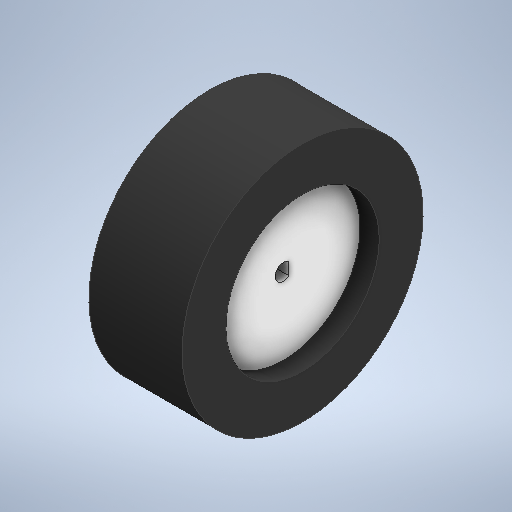
# Autodesk Inventor part: llanta
Saved by Autodesk Inventor 2025.2 (Build 292293000, 293)
## iProperties
Created: 2025-06-11
Part Number: llanta
Material: Generic
Document SubType Name: Modeling
Designer: cdavi
Density: 1 g/cm^3
Appearance: Default
Author: cdavi
Autodesk Inventor part; units mm, degrees
ref_plane "YZ Plane" through (0, 0, 0) normal (1, 0, 0) x (0, 1, 0)
ref_plane "XZ Plane" through (0, 0, 0) normal (0, 1, 0) x (-1, 0, 0)
ref_plane "XY Plane" through (0, 0, 0) normal (0, 0, 1) x (1, 0, 0)
sketch "Sketch1" plane through (0, 0, 0) normal (1, 0, 0) x (0, 1, 0)
  circle A0 centre (0, 0) radius 22
  circle A1 centre (0, 0) radius 14
  dimension "d0" = 44
  dimension "d1" = 8
  constraints: 2 centre point, 2 coincident
  measures "d0" diameter of A0
  measures "d1" radial gap between concentric circles of A1 A0
extrude "Extrusion1" add sketch "Sketch1" along normal blind 17
extrude "Extrusion2" add sketch "Sketch1" along normal blind 13.5 separate body contours A1
sketch "Sketch2" plane through (0, 0, 0) normal (-1, 0, 0) x (0, 0, 1)
  circle A0 centre (0, 0) radius 11
  circle A1 centre (0, 0) radius 13
  circle A2 centre (0, 0) radius 14 projected
  line L0 (0, 0) -> (2.2574, 12.8025) construction
  line L1 (0, 0) -> (0, 13)
  line L2 (0, 0) -> (-2.2574, 12.8025) construction
  line L3 (-2.2574, 12.8025) -> (-1.9101, 10.8329)
  line L4 (1.9101, 10.8329) -> (2.2574, 12.8025)
  line L5 (-3.7622, 10.3366) -> (-4.4463, 12.216)
  line L6 (-8.3562, 9.9586) -> (-7.0707, 8.4265)
  line L7 (-8.4265, 7.0707) -> (-9.9586, 8.3562)
  line L8 (-12.216, 4.4463) -> (-10.3366, 3.7622)
  line L9 (-10.8329, 1.9101) -> (-12.8025, 2.2574)
  line L10 (-12.8025, -2.2574) -> (-10.8329, -1.9101)
  line L11 (-10.3366, -3.7622) -> (-12.216, -4.4463)
  line L12 (-9.9586, -8.3562) -> (-8.4265, -7.0707)
  line L13 (-7.0707, -8.4265) -> (-8.3562, -9.9586)
  line L14 (-4.4463, -12.216) -> (-3.7622, -10.3366)
  line L15 (-1.9101, -10.8329) -> (-2.2574, -12.8025)
  line L16 (2.2574, -12.8025) -> (1.9101, -10.8329)
  line L17 (3.7622, -10.3366) -> (4.4463, -12.216)
  line L18 (8.3562, -9.9586) -> (7.0707, -8.4265)
  line L19 (8.4265, -7.0707) -> (9.9586, -8.3562)
  line L20 (12.216, -4.4463) -> (10.3366, -3.7622)
  line L21 (10.8329, -1.9101) -> (12.8025, -2.2574)
  line L22 (12.8025, 2.2574) -> (10.8329, 1.9101)
  line L23 (10.3366, 3.7622) -> (12.216, 4.4463)
  line L24 (9.9586, 8.3562) -> (8.4265, 7.0707)
  line L25 (7.0707, 8.4265) -> (8.3562, 9.9586)
  line L26 (4.4463, 12.216) -> (3.7622, 10.3366)
  point P0 (-4.4463, 12.216)
  point P1 (-3.7622, 10.3366)
  point P2 (-7.0707, 8.4265)
  point P3 (-8.4265, 7.0707)
  point P4 (-10.3366, 3.7622)
  point P5 (-12.216, 4.4463)
  point P6 (-12.8025, 2.2574)
  point P7 (-10.8329, 1.9101)
  point P8 (-10.8329, -1.9101)
  point P9 (-12.216, -4.4463)
  point P10 (-10.3366, -3.7622)
  point P11 (-8.4265, -7.0707)
  point P12 (-9.9586, -8.3562)
  point P13 (-8.3562, -9.9586)
  point P14 (-7.0707, -8.4265)
  point P15 (-3.7622, -10.3366)
  point P16 (-1.9101, -10.8329)
  point P17 (1.9101, -10.8329)
  point P18 (2.2574, -12.8025)
  point P19 (4.4463, -12.216)
  point P20 (7.0707, -8.4265)
  point P21 (8.3562, -9.9586)
  point P22 (9.9586, -8.3562)
  point P23 (8.4265, -7.0707)
  point P24 (10.3366, -3.7622)
  point P25 (12.216, -4.4463)
  point P26 (12.8025, -2.2574)
  point P27 (10.8329, -1.9101)
  point P28 (10.8329, 1.9101)
  point P29 (12.216, 4.4463)
  point P30 (8.4265, 7.0707)
  point P31 (9.9586, 8.3562)
  point P32 (8.3562, 9.9586)
  point P33 (3.7622, 10.3366)
  dimension "d7" = 2
  dimension "d6" = 1
  dimension "d8" = 10
  dimension "d9" = 3.8203
  dimension "d12" = 360
  constraints: 54 end point, 2 coincident, 2 point on line, 1 collinear, 1 symmetric about line, 1 vertical, 81 other
  measures "d8" angle of L1 L0
  measures "d9" distance of L4.start L3.end
extrude "Extrusion3" cut sketch "Sketch2" against normal blind 8 contours A0 | A0 L23 A1 L22 | L21 A1 L20 A0 | A0 L25 A1 L24 | L19 A1 L18 A0 | A0 L4 A1 L26 | L17 A1 L16 A0 | L15 A1 L14 A0 | A0 L5 A1 L3 | L13 A1 L12 A0 | A0 L7 A1 L6 | L11 A1 L10 A0 | A0 L9 A1 L8 | A2 bodies 2
sketch "Sketch3" plane through (13.5, 0, 0) normal (1, 0, 0) x (0, 0, -1)
  circle A0 centre (0, 0) radius 1.5
  line L0 (1, 1.118) -> (1, -1.118)
  dimension "d16" = 3
  dimension "d17" = 1
  constraints: 2 end point, 2 point on circle, 1 centre point, 1 coincident, 1 vertical
  measures "d16" diameter of A0
  measures "d17" distance from line of L0 A0.centre
extrude "Extrusion4" cut sketch "Sketch3" against normal through all contours L0 A0 picked at (0.1703, -0.0604) bodies 2
body "Solid1"
body "Solid2"
